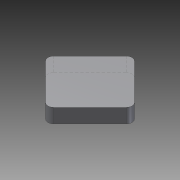
# Autodesk Inventor part: MatingPlates
Saved by Autodesk Inventor 2011 SP2 (Build 150309200, 309)
## iProperties
Created: 2014-05-12
Part Number: MatingPlates
Document SubType Name: Modeling
Designer: Maurice Woods
Density: 1 g/cm^3
Author: Maurice Woods
Autodesk Inventor part; units mm, degrees
ref_plane "YZ Plane" through (0, 0, 0) normal (1, 0, 0) x (0, 1, 0)
ref_plane "XZ Plane" through (0, 0, 0) normal (0, 1, 0) x (-1, 0, 0)
ref_plane "XY Plane" through (0, 0, 0) normal (0, 0, 1) x (1, 0, 0)
sketch "Sketch1" plane through (0, 0, 0) normal (0, 0, 1) x (1, 0, 0)
  line L0 (0, 25.4) -> (-25.4, 0) construction
  line L1 (-25.4, 0) -> (0, -25.4) construction
  line L2 (0, -25.4) -> (25.4, 0) construction
  line L3 (25.4, 0) -> (0, 25.4) construction
  line L4 (0, 25.4) -> (0, -25.4) construction
  line L5 (-25.4, 0) -> (25.4, 0) construction
  line L6 (-28.2284, 2.8284) -> (-2.8284, 28.2284)
  line L7 (2.8284, 28.2284) -> (28.2284, 2.8284)
  line L8 (28.2284, -2.8284) -> (2.8284, -28.2284)
  line L9 (-2.8284, -28.2284) -> (-28.2284, -2.8284)
  arc A0 (2.8284, 28.2284) -> (-2.8284, 28.2284) centre (0, 25.4) ccw
  arc A1 (28.2284, -2.8284) -> (28.2284, 2.8284) centre (25.4, 0) ccw
  arc A2 (-2.8284, -28.2284) -> (2.8284, -28.2284) centre (0, -25.4) ccw
  arc A3 (-28.2284, 2.8284) -> (-28.2284, -2.8284) centre (-25.4, 0) ccw
  point P0 (0, 0)
  point P1 (0, 0)
  dimension "d0" = 4
  dimension "d1" = 4
  dimension "d2" = 25.4
  constraints: 20 end point, 8 point on circle, 8 tangent, 4 centre point, 4 parallel, 3 equal radius, 3 perpendicular, 1 coincident, 1 midpoint, 1 vertical, 3 other
  measures "d0" distance between parallel lines of L8 L2
  measures "d1" radius of A0
  measures "d2" distance of point (0, 0) L0.end
extrude "Extrusion1" add sketch "Sketch1" along normal blind 5
sketch "Sketch2" plane through (0, 0, 5) normal (0, 0, 1) x (1, 0, 0)
  arc A0 (28.2284, -2.8284) -> (28.2284, 2.8284) centre (25.4, 0) ccw projected
  arc A1 (2.8284, 28.2284) -> (-2.8284, 28.2284) centre (0, 25.4) ccw projected
  arc A2 (-28.2284, 2.8284) -> (-28.2284, -2.8284) centre (-25.4, 0) ccw projected
  arc A3 (-2.8284, -28.2284) -> (2.8284, -28.2284) centre (0, -25.4) ccw projected
  point P0 (0, 0)
hole "Hole1" at (0, 25.4, 5) at (-25.4, 0, 5) at (0, -25.4, 5) at (25.4, 0, 5) at (0, 0, 5) direction (0, 0, -1) diameter 3.4 end through all clearance for "Socket Head Cap Screw" size "M3" standard "Ansi Metric M Profile"
equation "\"d2\" = LengthA"
equation "\"LengthA\" = 25.4"
body "Solid1"
